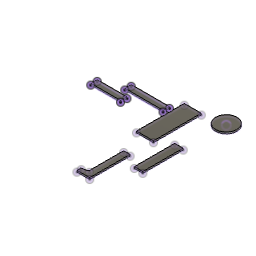
sisyphus (Autodesk Fusion 360 design; units mm, degrees)
Autodesk Fusion 360 part; units mm, degrees
note: some values were not read from the file. Set by a fixed rule: which sketch regions a step uses.
sketch "Sketch1" plane through (0, 0, 0) normal (0, 0, 1) x (1, 0, 0)
  line L0 (0, 0) -> (0, 95)
  line L1 (50, 75) -> (50, 170)
  line L2 (0, 0) -> (-30, 0)
  line L3 (-30, 0) -> (-30, 10)
  line L4 (0, 95) -> (-15, 95)
  line L5 (-15, 95) -> (-15, 14.2902)
  spline S0 degree 5 poles (-15, 14.2902) (-15.0922, 14.1253) (-15.2968, 13.8033) (-15.6637, 13.3431) (-16.2753, 12.776) (-17.255, 12.149) (-18.4623, 11.6086) (-19.9018, 11.1566) (-21.5597, 10.7877) (-23.4146, 10.4937) (-25.4445, 10.2662) (-27.1941, 10.1321) (-28.5719, 10.0565) (-29.5192, 10.017) (-30, 10) knots 0 0 0 0 0 0 0.1 0.2 0.3 0.4 0.5 0.6 0.7 0.8 0.9 1 1 1 1 1 1
  line L6 (50, 75) -> (30, 75)
  line L7 (30, 75) -> (30, 170)
  line L8 (30, 170) -> (50, 170)
  line L9 (0, 150) -> (0, 262.5)
  line L10 (0, 262.5) -> (-40, 262.5)
  line L11 (-40, 262.5) -> (-40, 150)
  line L12 (-40, 150) -> (0, 150)
  line L13 (50, 300) -> (50, 242.5)
  circle A0 centre (50, 271.25) radius 25
  point P0 (-18.4561, 11.6549)
  dimension "d8" = 95
  dimension "d9" = 95
  dimension "d10" = 30
  dimension "d11" = 15
  dimension "d12" = 112.5
  dimension "d13" = 57.5
  dimension "d14" = 50
  constraint coincident L0.start L2.start
  constraint vertical L1
  constraint perpendicular L0 L2
  constraint perpendicular L2 L3
  constraint perpendicular L0 L4
  constraint perpendicular L4 L5
  constraint perpendicular L1 L6
  constraint perpendicular L6 L7
  constraint perpendicular L1 L8
  constraint vertical L9
  constraint perpendicular L9 L10
  constraint perpendicular L10 L11
  constraint perpendicular L9 L12
  constraint vertical L13
  constraint midpoint L13 A0.centre
  measures "d8" distance of L0.start L0.end
  measures "d9" distance of L1.start L1.end
  measures "d10" distance of L0.start L2.end
  measures "d11" distance of L0.end L4.end
  measures "d12" distance of L9.start L9.end
  measures "d13" distance of L13.start L13.end
  measures "d14" diameter of A0
extrude "Extrude1" add sketch "Sketch1" along normal blind 3.8 makes body 1 at (42.4919, 267.6343, 3.8) makes body 2 at (43.3333, 106.6667, 0) makes body 3 at (-13.3333, 187.5, 0) makes body 4 at (-5, 36.4301, 0)
sketch "Sketch2" plane through (0, 0, 0) normal (0, 0, 1) x (1, 0, 0)
  line L0 (-40, 150) -> (0, 150)
  line L1 (0, 150) -> (0, 262.5)
  line L2 (0, 262.5) -> (-40, 262.5)
  line L3 (-40, 262.5) -> (-40, 150)
  circle A0 centre (50, 271.25) radius 25
  line L4 (50, 75) -> (50, 170)
  line L5 (50, 170) -> (30, 170)
  line L6 (30, 170) -> (30, 75)
  line L7 (30, 75) -> (50, 75)
  line L8 (0, 0) -> (0, 95)
  line L9 (0, 95) -> (-15, 95)
  line L10 (-15, 95) -> (-15, 14.2902)
  spline S0 degree 5 poles (-15, 14.2902) (-15.0922, 14.1253) (-15.2968, 13.8033) (-15.6637, 13.3431) (-16.2753, 12.776) (-17.255, 12.149) (-18.4623, 11.6086) (-19.9018, 11.1566) (-21.5597, 10.7877) (-23.4146, 10.4937) (-25.4445, 10.2662) (-27.1941, 10.1321) (-28.5719, 10.0565) (-29.5192, 10.017) (-30, 10) knots 0 0 0 0 0 0 0.1 0.2 0.3 0.4 0.5 0.6 0.7 0.8 0.9 1 1 1 1 1 1
  line L11 (-30, 10) -> (-30, 0)
  line L12 (-30, 0) -> (0, 0)
sketch "Sketch3" plane through (0, 0, 0) normal (0, 0, 1) x (1, 0, 0)
  line L0 (-100, 230) -> (-190, 230)
  line L1 (-190, 230) -> (-190, 215)
  line L2 (-190, 215) -> (-100, 215)
  line L3 (-100, 215) -> (-100, 230)
  line L4 (-170, 200) -> (-170, 185)
  line L5 (-170, 185) -> (-240, 185)
  line L6 (-240, 185) -> (-240, 200)
  line L7 (-240, 200) -> (-170, 200)
  dimension "d17" = 15
  dimension "d18" = 15
  dimension "d19" = 90
  dimension "d20" = 70
  constraint horizontal L0
  constraint perpendicular L0 L1
  constraint perpendicular L1 L2
  constraint perpendicular L0 L3
  constraint perpendicular L2 L4
  constraint perpendicular L4 L5
  constraint perpendicular L5 L6
  constraint perpendicular L4 L7
  measures "d17" distance of L0.end L1.end
  measures "d18" distance of L4.start L4.end
  measures "d19" distance of L0.start L0.end
  measures "d20" distance of L4.end L5.end
extrude "Extrude2" add sketch "Sketch3" along normal blind 3.8 separate body makes body 5 at (-160, 225, 0) makes body 6 at (-216.6667, 190, 0)
move_body "Move1" bodies 5 6 to x (1, 0, 0) y (0, 1, 0) z (0, 0, 1) at (48.9303, 8.6348, 0)
sketch "Sketch4" plane through (0, 0, 0) normal (0, 0, 1) x (1, 0, 0)
  line L0 (-51.0697, 223.6348) -> (-51.0697, 238.6348)
  line L1 (-51.0697, 238.6348) -> (-141.0697, 238.6348)
  line L2 (-141.0697, 238.6348) -> (-141.0697, 223.6348)
  line L3 (-141.0697, 223.6348) -> (-51.0697, 223.6348)
  line L4 (-191.0697, 208.6348) -> (-191.0697, 193.6348)
  line L5 (-191.0697, 193.6348) -> (-121.0697, 193.6348)
  line L6 (-121.0697, 193.6348) -> (-121.0697, 208.6348)
  line L7 (-121.0697, 208.6348) -> (-191.0697, 208.6348)
equation "overall_model_length = 300 mm"
equation "lower_leg_length = 75 mm"
equation "upper_leg_length = 75 mm"
equation "torso_length = 112.5 mm"
equation "head_length = 37.5 mm"
equation "joint = 20 mm"
equation "d8 = lower_leg_length + joint"
equation "d9 = upper_leg_length + joint"
equation "d12 = torso_length"
equation "d13 = head_length + joint"
